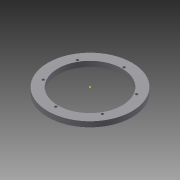
# Autodesk Inventor part: middle plate
Saved by Autodesk Inventor 2015 (Build 190159000, 159)
## iProperties
Created: 2015-02-28
Part Number: middle plate
Material: Generic
Document SubType Name: Modeling
Designer: Qiuyang
Density: 1 g/cm^3
Appearance: Default
Author: Qiuyang
Autodesk Inventor part; units mm, degrees
ref_plane "YZ Plane" through (0, 0, 0) normal (1, 0, 0) x (0, 1, 0)
ref_plane "XZ Plane" through (0, 0, 0) normal (0, 1, 0) x (-1, 0, 0)
ref_plane "XY Plane" through (0, 0, 0) normal (0, 0, 1) x (1, 0, 0)
sketch "Sketch1" plane through (0, 0, 0) normal (0, 1, 0) x (-1, 0, 0)
  circle A0 centre (0, 0) radius 38.735
  circle A1 centre (0, 0) radius 50.8
  circle A2 centre (0, 41.275) radius 1.524
  circle A3 centre (-35.7452, 20.6375) radius 1.524
  circle A4 centre (-35.7452, -20.6375) radius 1.524
  circle A5 centre (0, -41.275) radius 1.524
  circle A6 centre (35.7452, -20.6375) radius 1.524
  circle A7 centre (35.7452, 20.6375) radius 1.524
  dimension "d0" = 77.47
  dimension "d1" = 101.6
  dimension "d2" = 3.048
  dimension "d5" = 360
  constraints: 9 coincident, 8 centre point, 23 other
  measures "d0" diameter of A0
  measures "d1" diameter of A1
  measures "d2" diameter of A2
extrude "Extrusion1" add sketch "Sketch1" along normal blind 6.35
sketch "Sketch2" plane through (0, 6.35, 0) normal (0, 1, 0) x (1, 0, 0)
  point P0 (0, 0)
sketch "Sketch3" plane through (0, 6.35, 0) normal (0, 1, 0) x (1, 0, 0)
  point P0 (0, 0)
body "Solid1"
